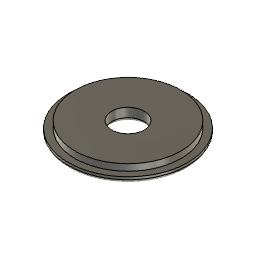
vial_adapter_screw_no4 (Autodesk Fusion 360 design; units mm, degrees)
Autodesk Fusion 360 part; units mm, degrees
sketch "スケッチ1" plane through (0, 0, 0) normal (0, 0, 1) x (1, 0, 0)
  circle A0 centre (0, 0) radius 46
  dimension "d1" = 92
  constraint coincident A0.centre origin
  measures "d1" diameter of A0
extrude "押し出し1" add sketch "スケッチ1" along normal blind 10
sketch "スケッチ2" plane through (0, 0, 10) normal (0, 0, 1) x (-1, 0, 0)
  circle A0 centre (0, 0) radius 46
  circle A1 centre (0, 0) radius 40.75
  dimension "d4" = 81.5
  constraint coincident A0.centre A1.centre
  measures "d4" diameter of A1
extrude "押し出し2" cut sketch "スケッチ2" against normal blind 5
sketch "スケッチ3" plane through (0, 0, 10) normal (0, 0, 1) x (-1, 0, 0)
  circle A0 centre (0, 0) radius 40.75
  circle A1 centre (0, 0) radius 12.5
  dimension "d7" = 25
  constraint coincident A0.centre A1.centre
  measures "d7" diameter of A1
extrude "押し出し3" cut sketch "スケッチ3" against normal blind 10 contours A1
fillet "フィレット1" radius 3 1 faces at (34.6155, -2.9063, 0)
